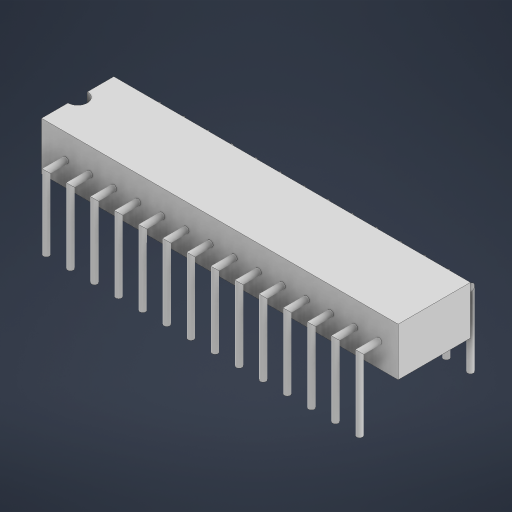
# Autodesk Inventor part: Part3
Saved by Autodesk Inventor 2024 (Build 280153000, 153)
## iProperties
Created: 2023-12-19
Part Number: Part3
Material: Generic
Document SubType Name: Sheet Metal
Designer: Shado
Density: 1 g/cm^3
Sheet Metal Rule: Default
Appearance: Default
Author: Shado
Autodesk Inventor part; units mm, degrees
ref_plane "YZ Plane" through (0, 0, 0) normal (1, 0, 0) x (0, 1, 0)
ref_plane "XZ Plane" through (0, 0, 0) normal (0, 1, 0) x (-1, 0, 0)
ref_plane "XY Plane" through (0, 0, 0) normal (0, 0, 1) x (1, 0, 0)
sketch "Sketch1" plane through (0, 0, 0) normal (0, 1, 0) x (-1, 0, 0)
  line L0 (0, 0) -> (37, 0)
  line L1 (37, -7.5) -> (0, -7.5)
  line L2 (0, -7.5) -> (0, 0)
  arc A0 (37, -2.75) -> (37, -4.75) centre (37, -3.75) ccw
  line L3 (37, 0) -> (37, -2.75)
  line L4 (37, -4.75) -> (37, -7.5)
  dimension "d0" = 37
  dimension "d1" = 7.5
  dimension "d2" = 2
  constraints: 10 end point, 3 parallel, 2 perpendicular, 2 point on circle, 1 centre point, 1 horizontal
  measures "d0" distance of L1.start L1.end
  measures "d1" distance of L0.end L1.start
  measures "d2" diameter of A0
extrude "Extrusion1" add sketch "Sketch1" along normal blind 5
sketch "Sketch2" plane through (-37, 0, 0) normal (0, 0, 1) x (1, 0, 0)
  circle A0 centre (2.5, 2.5) radius 0.3
  circle A1 centre (5, 2.5) radius 0.3
  circle A2 centre (7.5, 2.5) radius 0.3
  circle A3 centre (10, 2.5) radius 0.3
  circle A4 centre (12.5, 2.5) radius 0.3
  circle A5 centre (15, 2.5) radius 0.3
  circle A6 centre (17.5, 2.5) radius 0.3
  circle A7 centre (20, 2.5) radius 0.3
  circle A8 centre (22.5, 2.5) radius 0.3
  circle A9 centre (25, 2.5) radius 0.3
  circle A10 centre (27.5, 2.5) radius 0.3
  circle A11 centre (30, 2.5) radius 0.3
  circle A12 centre (32.5, 2.5) radius 0.3
  circle A13 centre (35, 2.5) radius 0.3
  point P0 (37, 0)
  dimension "d5" = 0.6
  dimension "d7" = 0.6
  dimension "d8" = 0.6
  dimension "d9" = 0.6
  dimension "d11" = 0.6
  dimension "d12" = 0.6
  dimension "d13" = 0.6
  dimension "d14" = 0.6
  dimension "d15" = 0.6
  dimension "d16" = 0.6
  dimension "d17" = 0.6
  dimension "d18" = 0.6
  dimension "d19" = 0.6
  dimension "d20" = 0.6
  constraints: 14 centre point
  measures "d5" diameter of A0
  measures "d7" diameter of A1
  measures "d8" diameter of A2
  measures "d9" diameter of A3
  measures "d11" diameter of A4
  measures "d12" diameter of A5
  measures "d13" diameter of A6
  measures "d14" diameter of A7
  measures "d15" diameter of A8
  measures "d16" diameter of A9
  measures "d17" diameter of A10
  measures "d18" diameter of A11
  measures "d19" diameter of A12
  measures "d20" diameter of A13
sketch3d "3D Sketch1"
  line L0 (-2, 2.5, 0) -> (-2, 2.5, 2)
  line L1 (-2, 2.5, 2) -> (-2, -5, 2)
  dimension "d23" = 2
  dimension "d24" = 7.5
sweep "Sweep1" add profiles "Sketch2" path "3D Sketch1"
sketch "Sketch3" plane through (0, 0, -7.5) normal (0, 0, -1) x (-1, 0, 0)
  arc A0 (2.3, 2.5) -> (1.7, 2.5) centre (2, 2.5) ccw projected
  circle A1 centre (2, 2.5) radius 0.3
  arc A2 (4.8, 2.5) -> (4.2, 2.5) centre (4.5, 2.5) ccw projected
  circle A3 centre (4.5, 2.5) radius 0.3
  circle A4 centre (7, 2.5) radius 0.3 projected
  circle A5 centre (7, 2.5) radius 0.3
  circle A6 centre (9.5, 2.5) radius 0.3 projected
  circle A7 centre (9.5, 2.5) radius 0.3
  circle A8 centre (12, 2.5) radius 0.3 projected
  circle A9 centre (12, 2.5) radius 0.3
  arc A10 (14.2, 2.5) -> (14.8, 2.5) centre (14.5, 2.5) ccw projected
  circle A11 centre (14.5, 2.5) radius 0.3
  circle A12 centre (17, 2.5) radius 0.3 projected
  circle A13 centre (17, 2.5) radius 0.3
  circle A14 centre (19.5, 2.5) radius 0.3 projected
  circle A15 centre (19.5, 2.5) radius 0.3
  circle A16 centre (22, 2.5) radius 0.3 projected
  circle A17 centre (22, 2.5) radius 0.3
  circle A18 centre (24.5, 2.5) radius 0.3 projected
  circle A19 centre (24.5, 2.5) radius 0.3
  circle A20 centre (29.5, 2.5) radius 0.3 projected
  circle A21 centre (29.5, 2.5) radius 0.3
  circle A22 centre (27, 2.5) radius 0.3 projected
  circle A23 centre (27, 2.5) radius 0.3
  circle A24 centre (32, 2.5) radius 0.3 projected
  circle A25 centre (32, 2.5) radius 0.3
  circle A26 centre (34.5, 2.5) radius 0.3 projected
  circle A27 centre (34.5, 2.5) radius 0.3
  point P0 (0, 0)
  constraints: 14 centre point, 14 coincident
sketch3d "3D Sketch2"
  line L0 (-2, 2.5, -7.5) -> (-2, 2.5, -9.5)
  line L1 (-2, 2.5, -9.5) -> (-2, -5, -9.5)
  dimension "d27" = 2
  dimension "d28" = 7.5
sweep "Sweep2" add profiles "Sketch3" path "3D Sketch2"
equation "\"BendRadius\" = Thickness"
equation "\"BendReliefWidth\" = Thickness"
equation "\"BendReliefDepth\" = 0.5 * Thickness"
equation "\"CornerReliefSize\" = 4 * Thickness"
equation "\"MinimumRemnant\" = 2 * Thickness"
equation "\"TransitionRadius\" = BendRadius"
equation "\"JacobiRadiusSize\" = BendRadius"
equation "\"GapSize\" = Thickness"
equation "\"Thickness\" = 3.048"
body "Solid1"
